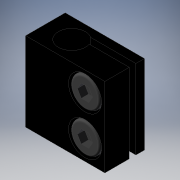
# Autodesk Inventor part: SCHUNK-9700901 Halter fuer NHS Du 4
Saved by Autodesk Inventor 2019 (Build 230136000, 136)
## iProperties
Created: 2022-08-29
Part Number: SCHUNK-9700901 Halter fuer NHS Du 4
Material: Generic
Catalog Web Link: www.cadenas.de
Description: Halterung für Nährungsschalter-MPGplus
Vendor: SCHUNK
Document SubType Name: Modeling
Designer: psAdmin
Manufacturer: SCHUNK
Mass: 0.620229 g
Surface Area: 10.7575 cm^2
Volume: 0.620229 cm^3
Density: 1 g/cm^3
Appearance: PSOLRGB-0-0-0
Category: PARTsolutions
Company: SCHUNK
Title: SCHUNK-9700901 Halter fuer NHS Du 4
Author: Cadenas PARTsolutions
Comments: MPGplus
PSOL_IDENT_0: {$CADENAS_DATA/23d-libs/schunk/greifsysteme/greifmodule/greifmodule_pneumatisch/2_finger_parallelgre
PSOL_IDENT_1: ifer/2_finger_kleinteilegreifer/mpg_plus/mpgplus_hal_as.prj},234 {VTYP=3D},{NB=SCHUNK-9700901 Halter
PSOL_IDENT_2: fuer NHS Du 4},{LINA=SCHUNK-9700901 Halter fuer NHS Du 4},{NN=Halterung für Nährungsschalter},{DATE=
PSOL_IDENT_3: 23.03.2022 14:50:11},{GEOMDATE=15.04.2020 08:38:32},{VERSION=},{LINEID=20},{WBVAR=},{WBNUMERIC=}  {N
PSOL_IDENT_4: B=SCHUNK-9700901 Halter fuer NHS Du 4},{LINA=SCHUNK-9700901 Halter fuer NHS Du 4},{KT=DUMMY},{IDNR=9
PSOL_IDENT_5: 700901},{TYP=Halter fuer NHS Du 4},{TYP1=2.000},{L=12.000},{L1=9.000},{L2=4.000},{B=6.000},{B1=3.000
PSOL_IDENT_6: },{B2=1.300},{B3=1.000},{H=12.000},{H1=3.000},{H2=6.000},{D1=4.100},{D2=2.800},{D3=5.000},{DT3=2.500
PSOL_IDENT_7: },{DSK=4.500},{HSK=2.500},{LGS=5.000},{GS=2.500},{SWS=2.000},{TSWS=1.100},{CNSCTN=84799070}
NB: SCHUNK-9700901 Halter fuer NHS Du 4
NN: Halterung für Nährungsschalter
NT: MPGplus
NBSYN: SCHUNK-$IDNR. $TYP.
LINA: SCHUNK-9700901 Halter fuer NHS Du 4
CATALOG: SCHUNK
IDNR: 9700901
TYP: Halter fuer NHS Du 4
TYP1: 2
L: 12
L1: 9
L2: 4
B: 6
B1: 3
B2: 1.3
B3: 1
H: 12
H1: 3
H2: 6
D1: 4.1
D2: 2.8
D3: 5
DT3: 2.5
DSK: 4.5
HSK: 2.5
LGS: 5
GS: 2.5
SWS: 2
TSWS: 1.1
CNSCTN: 84799070
SUPPLIER: SCHUNK
ARTICLENO: SCHUNK-9700901 Halter fuer NHS Du 4
BOMINFO: SCHUNK-9700901 Halter fuer NHS Du 4
CREATOR: CADENAS GmbH
Autodesk Inventor part; units mm, degrees
sketch "Sketch_1" plane through (0, 0, 0) normal (0, 1, 0) x (-1, 0, 0)
  line L0 (0, 6) -> (-12, 6)
  line L1 (-12, 6) -> (-12, 2.3)
  line L2 (-12, 2.3) -> (-5.9268, 2.3)
  arc A0 (-5.1456, 1.3) -> (-5.9268, 2.3) centre (-4, 3) ccw
  line L3 (-5.1456, 1.3) -> (-12, 1.3)
  line L4 (-12, 1.3) -> (-12, 0)
  line L5 (-12, 0) -> (0, 0)
  line L6 (0, 0) -> (0, 6)
  constraints: 14 end point, 2 point on circle, 1 centre point
extrude "Extrusion1" add sketch "Sketch_1" along normal blind 12
sketch "Sketch2" plane through (12, 0, 0) normal (0, 0, -1) x (-1, 0, 0)
  point P0 (3, 3)
hole "Hole1" at (9, 3, 0) direction (0, 0, 1) diameter 2.8 depth 6
pattern_linear "Rectangular Pattern1" count 2 spacing 6 along (0, 1, 0) of "Hole1"
sketch "Sketch_4" plane through (9, 0, 0) normal (1, 0, 0) x (0, 0, -1)
  line L0 (-3.5, 3) -> (-6, 3)
  line L1 (-6, 3) -> (-6, 5.5)
  line L2 (-6, 5.5) -> (-3.5, 5.5)
  line L3 (-3.5, 5.5) -> (-3.5, 3)
  line L4 (-3.5, 3) -> (-6, 3)
  constraints: 10 end point
revolve "Revolution1" cut sketch "Sketch_4" angle 360 about axis through (9, 3, 3.5) along (0, 0, -1)
pattern_linear "Rectangular Pattern2" count 2 spacing 6 along (0, 1, 0) of "Revolution1"
sketch "Sketch_12" plane through (9, 0, 0) normal (1, 0, 0) x (0, 0, -1)
  line L0 (1.5, 3) -> (-6, 3)
  line L1 (-6, 3) -> (-6, 4.95)
  arc A0 (-5.7, 5.25) -> (-6, 4.95) centre (-5.7, 4.95) ccw
  line L2 (-5.7, 5.25) -> (-3.5, 5.25)
  line L3 (-3.5, 5.25) -> (-3.5, 4.25)
  line L4 (-3.5, 4.25) -> (1.3, 4.25)
  line L5 (1.3, 4.25) -> (1.5, 4.05)
  line L6 (1.5, 4.05) -> (1.5, 3)
  line L7 (1.5, 3) -> (-6, 3)
  constraints: 16 end point, 2 point on circle, 1 centre point
revolve "Revolution2" add sketch "Sketch_12" angle 360 about axis through (9, 3, -1.5) along (0, 0, -1)
thread "Thread1" size "M2.5x0.45" class "6g" standard "ISO Metric profile" full length
pattern_linear "Rectangular Pattern3" count 2 spacing 6 along (0, 1, 0) of "Revolution2"
sketch "Sketch_14" plane through (9, 3, 6) normal (0, 0, 1) x (0, 1, 0)
  line L0 (-1, -0.5774) -> (0, -1.1547)
  line L1 (0, -1.1547) -> (1, -0.5774)
  line L2 (1, -0.5774) -> (1, 0.5774)
  line L3 (1, 0.5774) -> (0, 1.1547)
  line L4 (0, 1.1547) -> (-1, 0.5774)
  line L5 (-1, 0.5774) -> (-1, -0.5774)
  constraints: 12 end point
extrude "Extrusion2" cut sketch "Sketch_14" against normal blind 1.1
pattern_linear "Rectangular Pattern4" count 2 spacing 6 along (0, 1, 0) of "Extrusion2"
ref_plane "as_nhs_01_XY" through (9, 3, 0) normal (0, 0, 1) x (1, 0, 0)
ref_plane "as_nhs_01_YZ" through (9, 3, 0) normal (1, 0, 0) x (0, 1, 0)
ref_plane "as_nhs_01_ZX" through (9, 3, 0) normal (0, 1, 0) x (0, 0, 1)
ref_plane "as_nhs_02_XY" through (9, 9, 0) normal (0, 0, 1) x (1, 0, 0)
ref_plane "as_nhs_02_YZ" through (9, 9, 0) normal (1, 0, 0) x (0, 1, 0)
ref_plane "as_nhs_02_ZX" through (9, 9, 0) normal (0, 1, 0) x (0, 0, 1)
ref_plane "s01_XY" through (9, 3, 3.5) normal (0, 0, 1) x (1, 0, 0)
ref_plane "s01_YZ" through (9, 3, 3.5) normal (1, 0, 0) x (0, 1, 0)
ref_plane "s01_ZX" through (9, 3, 3.5) normal (0, 1, 0) x (0, 0, 1)
ref_plane "s02_XY" through (9, 9, 3.5) normal (0, 0, 1) x (1, 0, 0)
ref_plane "s02_YZ" through (9, 9, 3.5) normal (1, 0, 0) x (0, 1, 0)
ref_plane "s02_ZX" through (9, 9, 3.5) normal (0, 1, 0) x (0, 0, 1)
body "Solid1"
